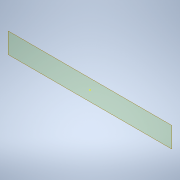
# Autodesk Inventor part: hinge
Saved by Autodesk Inventor 2021 (Build 250183000, 183)
## iProperties
Created: 2021-04-17
Part Number: hinge
Material: Generic
Document SubType Name: Modeling
Designer: gfellows
Density: 1 g/cm^3
Appearance: Default
Author: gfellows
Autodesk Inventor part; units mm, degrees
ref_plane "YZ Plane" through (0, 0, 0) normal (1, 0, 0) x (0, 1, 0)
ref_plane "XZ Plane" through (0, 0, 0) normal (0, 1, 0) x (-1, 0, 0)
ref_plane "XY Plane" through (0, 0, 0) normal (0, 0, 1) x (1, 0, 0)
ref_plane "Work Plane1" through (-192, 24, -212) normal (0, 0, -1) x (-1, 0, 0)
sketch "Sketch1" plane through (-192, 24, -212) normal (0, 0, -1) x (-1, 0, 0)
  circle A0 centre (-32, -8) radius 2 projected
  arc A1 (-30.5858, -33.4142) -> (-33.4142, -30.5858) centre (-32, -32) ccw projected
  arc A2 (-6.5858, -33.4142) -> (-9.4142, -30.5858) centre (-8, -32) ccw projected
  circle A3 centre (-8, -8) radius 2 projected
  circle A4 centre (-32, -32) radius 2
  circle A5 centre (-8, -32) radius 2
  circle A6 centre (-8, -8) radius 2
  circle A7 centre (-32, -8) radius 2
  circle A8 centre (-32, -8) radius 3
  circle A9 centre (-8, -8) radius 3
  circle A10 centre (-8, -32) radius 3
  circle A11 centre (-32, -32) radius 3
  line L0 (-35, -8) -> (-35, -32)
  line L1 (-32, -35) -> (-8, -35)
  line L2 (-5, -32) -> (-5, -8)
  line L3 (-8, -5) -> (-32, -5)
  point P0 (-192, -24)
  point P1 (-9.4142, -30.5858)
  point P2 (-33.4142, -30.5858)
  dimension "d0" = 1
  dimension "d1" = 1
  dimension "d2" = 1
  dimension "d3" = 1
  constraints: 8 end point, 8 point on circle, 7 tangent, 6 centre point, 4 coincident, 2 concentric, 1 vertical, 6 other
  measures "d0" radial gap between concentric circles of A0 A8
  measures "d1" radial gap between concentric circles of A3 A9
extrude "Extrusion1" add sketch "Sketch1" along normal blind 4
sketch "Sketch2" plane through (-192, 24, -216) normal (0, 0, -1) x (-1, 0, 0)
  line L0 (-35, -8) -> (-35, -32) projected
  line L1 (-5, -32) -> (-5, -8) projected
  line L2 (-5, -32) -> (-5, -8) projected
  line L3 (-35, -11) -> (-5, -11)
  line L4 (-5, -11) -> (-5, -29)
  line L5 (-5, -29) -> (-35, -29)
  line L6 (-35, -29) -> (-35, -11)
  circle A0 centre (-32, -8) radius 2 projected
  circle A1 centre (-8, -8) radius 2 projected
  circle A2 centre (-8, -32) radius 2 projected
  circle A3 centre (-32, -32) radius 2 projected
  line L7 (-29, -11) -> (-29, -29)
  line L8 (-11, -11) -> (-11, -29)
  point P0 (-192, -24)
  dimension "d6" = 3
  dimension "d7" = 3
  dimension "d8" = 3
  dimension "d9" = 3
  constraints: 12 end point, 6 point on line, 3 perpendicular, 2 parallel, 1 horizontal
  measures "d6" distance from line of L5 A3.centre
  measures "d7" distance from line of A0.centre L3
  measures "d8" distance from line of L8 A1.centre
  measures "d9" distance from line of L7 A0.centre
extrude "Extrusion2" add sketch "Sketch2" along normal blind 10 contours L3 L8 L5 L7
sketch "Sketch3" plane through (-181, -5, -216) normal (-1, 0, 0) x (0, 0, 1)
  line L0 (0, 18) -> (0, 0) projected
  line L1 (0, 18) -> (-10, 18) projected
  line L2 (-10, 0) -> (-10, 18) projected
  line L3 (0, 0) -> (-10, 0) projected
  line L4 (-10, 18) -> (-10, 0) projected
  line L5 (0, 21) -> (0, -3) projected
  line L6 (-10, 14) -> (0, 14)
  line L7 (0, 14) -> (0, 4)
  line L8 (0, 4) -> (-10, 4)
  line L9 (-10, 4) -> (-10, 14)
  point P0 (216, 5)
  point P1 (-10, 4)
  point P2 (0, 4)
  point P3 (0, 14)
  dimension "d12" = 4
  dimension "d13" = 4
  constraints: 8 end point, 2 parallel, 2 point on line, 1 horizontal, 1 perpendicular
  measures "d12" distance between parallel lines of L1 L6
  measures "d13" distance between parallel lines of L3 L8
extrude "Extrusion3" cut sketch "Sketch3" against normal through all contours L0 L8 L2 L6
fillet "Fillet1" radius 3.175 8 edges at (-181, 11, -226) (-163, 11, -226) (-181, 11, -216) (-163, 11, -216) (-163, -3, -216) (-163, -3, -226) (-181, -3, -226) (-181, -3, -216)
sketch "Sketch4" plane through (-184.175, 13, -216) normal (0, 1, 0) x (1, 0, 0)
  arc A0 (21.175, 6.825) -> (18, 10) centre (18, 6.825) ccw projected
  line L0 (6.35, 10) -> (18, 10) projected
  arc A1 (6.35, 10) -> (3.175, 6.825) centre (6.35, 6.825) ccw projected
  line L1 (3.175, 3.175) -> (3.175, 6.825) projected
  arc A2 (0, 0) -> (3.175, 3.175) centre (0, 3.175) ccw projected
  line L2 (24.35, 0) -> (0, 0) projected
  arc A3 (21.175, 3.175) -> (24.35, 0) centre (24.35, 3.175) ccw projected
  line L3 (21.175, 3.175) -> (21.175, 6.825) projected
  circle A4 centre (12.175, 5) radius 2
  point P0 (184.175, -216)
  dimension "d17" = 4
  dimension "d18" = 18
  dimension "d19" = 9
  dimension "d20" = 10
  dimension "d21" = 5
  constraints: 1 centre point
  measures "d17" diameter of A4
  measures "d18" distance between parallel lines of L1 L3
  measures "d19" distance from line of L1 A4.centre
  measures "d20" distance between parallel lines of L2 L0
  measures "d21" distance from line of L2 A4.centre
extrude "Extrusion4" cut sketch "Sketch4" against normal through all contours A4
equation "\"d19\" = 0.5 * d18"
equation "\"d21\" = 0.5 * d20"
body "Solid1"
